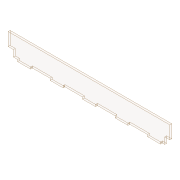
# Autodesk Inventor part: Divisória-24cm
Saved by Autodesk Inventor 2020 (Build 240168000, 168)
## iProperties
Created: 2021-09-22
Part Number: Divisória-24cm
Material: Generic
Document SubType Name: Modeling
Designer: pablo
Density: 1 g/cm^3
Appearance: Polycarbonate - Smoked
Author: pablo
Autodesk Inventor part; units mm, degrees
ref_plane "YZ Plane" through (0, 0, 0) normal (1, 0, 0) x (0, 1, 0)
ref_plane "XZ Plane" through (0, 0, 0) normal (0, 1, 0) x (-1, 0, 0)
ref_plane "XY Plane" through (0, 0, 0) normal (0, 0, 1) x (1, 0, 0)
sketch "Sketch1" plane through (0, 0, 0) normal (0, 0, 1) x (1, 0, 0)
  line L0 (-124.5, 15) -> (124.5, 15)
  line L1 (124.5, 15) -> (124.5, -15)
  line L2 (124.5, -15) -> (-124.5, -15)
  line L3 (-124.5, -15) -> (-124.5, 15)
  line L4 (-124.5, 15) -> (124.5, -15) construction
  line L5 (124.5, 15) -> (-124.5, -15) construction
  point P0 (0, 0)
  dimension "d0" = 30
  dimension "d1" = 249
  constraints: 12 end point, 2 midpoint, 2 parallel, 1 horizontal, 1 perpendicular
  measures "d0" distance of L0.end L1.end
  measures "d1" distance of L1.end L2.end
extrude "Extrusion1" add sketch "Sketch1" along normal blind 3
sketch "Sketch2" plane through (0, 0, 3) normal (0, 0, 1) x (1, 0, 0)
  line L0 (-110, -14.8732) -> (-90, -14.8732)
  line L1 (-90, -14.8732) -> (-90, -17.8732)
  line L2 (-90, -17.8732) -> (-110, -17.8732)
  line L3 (-110, -17.8732) -> (-110, -14.8732)
  line L4 (-124.5, 15) -> (-124.5, -15) projected
  line L5 (-60, -14.8732) -> (-40, -14.8732)
  line L6 (-40, -14.8732) -> (-40, -17.8732)
  line L7 (-40, -17.8732) -> (-60, -17.8732)
  line L8 (-60, -17.8732) -> (-60, -14.8732)
  line L9 (-10, -14.8732) -> (10, -14.8732)
  line L10 (10, -14.8732) -> (10, -17.8732)
  line L11 (10, -17.8732) -> (-10, -17.8732)
  line L12 (-10, -17.8732) -> (-10, -14.8732)
  line L13 (40, -14.8732) -> (60, -14.8732)
  line L14 (60, -14.8732) -> (60, -17.8732)
  line L15 (60, -17.8732) -> (40, -17.8732)
  line L16 (40, -17.8732) -> (40, -14.8732)
  line L17 (90, -14.8732) -> (110, -14.8732)
  line L18 (110, -14.8732) -> (110, -17.8732)
  line L19 (110, -17.8732) -> (90, -17.8732)
  line L20 (90, -17.8732) -> (90, -14.8732)
  line L21 (124.5, -15) -> (124.5, 15) projected
  point P0 (0, 0)
  dimension "d4" = 20
  dimension "d5" = 3
  dimension "d6" = 14.5
  dimension "d9" = 50
  dimension "d22" = 14.5
  constraints: 40 end point, 2 horizontal, 2 parallel, 1 collinear, 1 perpendicular, 31 other
  measures "d4" distance of L1.end L2.end
  measures "d5" distance of L0.end L1.end
  measures "d6" distance from line of L4 L0.start
  measures "d9" distance of L0.start L5.start
  measures "d22" distance from line of L18.end L21
extrude "Extrusion2" add sketch "Sketch2" against normal blind 3
sketch "Sketch3" plane through (0, 0, 3) normal (0, 0, 1) x (1, 0, 0)
  line L0 (-124.5, 15) -> (-124.5, -15) projected
  line L1 (-124.5, -15) -> (-116.5, -15)
  line L2 (-116.5, -15) -> (-116.5, -5)
  line L3 (-116.5, -5) -> (-124.5, -5)
  line L4 (-124.5, -5) -> (-124.5, -15)
  line L5 (0, 0) -> (0, -7.9678)
  line L6 (124.5, -15) -> (116.5, -15)
  line L7 (116.5, -15) -> (116.5, -5)
  line L8 (116.5, -5) -> (124.5, -5)
  line L9 (124.5, -5) -> (124.5, -15)
  dimension "d18" = 8
  dimension "d19" = 10
  constraints: 18 end point, 4 symmetric about line, 2 parallel, 1 horizontal, 1 perpendicular, 1 vertical
  measures "d18" distance of L3.end L2.end
  measures "d19" distance of L2.end L1.end
extrude "Extrusion3" cut sketch "Sketch3" against normal blind 3
body "Solid1"
